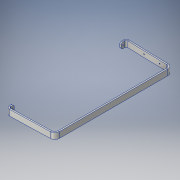
# Autodesk Inventor part: Panel_Strut
Saved by Autodesk Inventor 2016 (Build 200138000, 138)
## iProperties
Created: 2016-03-26
Part Number: Panel_Strut
Material: Aluminum 6061
Document SubType Name: Sheet Metal
Designer: agmle
Density: 2.7 g/cm^3
Sheet Metal Rule: Default
Appearance: Aluminum - Flat
Mass: 48.4378 g
Surface Area: 147.191 cm^2
Volume: 17.9399 cm^3
Flat Pattern Width: 1.27 cm
Flat Pattern Length: 46.2876 cm
Flat Pattern Area: 58.7853 cm^2
Sheet Metal Width: 0.500 in
Sheet Metal Length: 18.223 in
Sheet Metal Area: 9.112 in^2
Author: agmle
Autodesk Inventor part; units mm, degrees
ref_plane "YZ Plane" through (0, 0, 0) normal (1, 0, 0) x (0, 1, 0)
ref_plane "XZ Plane" through (0, 0, 0) normal (0, 1, 0) x (-1, 0, 0)
ref_plane "XY Plane" through (0, 0, 0) normal (0, 0, 1) x (1, 0, 0)
sketch "Sketch1" plane through (0, 0, 0) normal (0, 1, 0) x (-1, 0, 0)
  line L0 (110.8964, 130.0226) -> (9.5972, 127.37)
  line L1 (0, 117.5182) -> (0, -117.5182)
  line L2 (9.5972, -127.37) -> (110.8964, -130.0226)
  arc A0 (9.5972, 127.37) -> (0, 117.5182) centre (9.8552, 117.5182) ccw
  arc A1 (0, -117.5182) -> (9.5972, -127.37) centre (9.8552, -117.5182) ccw
  line L3 (110.8964, 130.0226) -> (0, 130.0226) construction
  line L4 (0, 130.0226) -> (0, -130.0226) construction
  line L5 (0, -130.0226) -> (110.8964, -130.0226) construction
  line L6 (110.8964, -130.0226) -> (110.8964, 130.0226) construction
  line L7 (102.7684, 130.0226) -> (102.7684, -130.0226) construction
  point P0 (0, 0)
  point P1 (0, 127.1187)
  point P2 (0, 0)
  dimension "d1" = 91.5
  dimension "d2" = 91.5
  dimension "d4" = 9.8552
  dimension "d15" = 260.0452
  dimension "d16" = 110.8964
  dimension "d17" = 8.128
  measures "d1" angle of L1 L0
  measures "d2" angle of L1 L2
  measures "d4" radius of A0
  measures "d15" distance of L5.end L3.start
  measures "d16" distance of L3.start L3.end
  measures "d17" distance between parallel lines of L6 L7
contour flange "Contour Flange1" sketch "Sketch1" thickness 3.048 bend radius 3.048 width 12.7 along (0, 1, 0) mid plane no both sides no wall seen from (-60.2468, 0, 128.6963) lies toward (-0.0261769, 0, -0.9996573) curves L0 A0 L1 A1 L2
bend "Bend1"
corner "Corner1"
sketch "Sketch2" plane through (-9.677, 0, 124.323) normal (-0.0261769, 0, -0.9996573) x (-0.9996573, 0, 0.0261769)
  line L0 (0, 0) -> (0, 12.7) construction
  line L1 (101.3339, 0) -> (0, 0) construction
  line L2 (101.3339, 12.7) -> (101.3339, 0) construction
  line L3 (0, 12.7) -> (101.3339, 12.7) construction
  line L4 (101.3339, 12.7) -> (0, 12.7) projected
  line L5 (90.1579, 12.7) -> (90.1579, 0)
  line L6 (101.3339, 0) -> (0, 0) projected
  point P0 (-12.9281, 0)
  dimension "d18" = 11.176
  constraints: 2 end point, 2 point on line, 1 perpendicular
  measures "d18" distance between parallel lines of L5 L2
sketch "Sketch3" plane through (-9.677, 0, -124.323) normal (-0.0261769, 0, 0.9996573) x (0.9996573, 0, 0.0261769)
  line L0 (0, 0) -> (0, 12.7) construction
  line L1 (-101.3339, 12.7) -> (0, 12.7) construction
  line L2 (-101.3339, 0) -> (-101.3339, 12.7) construction
  line L3 (0, 0) -> (-101.3339, 0) construction
  line L4 (-90.1579, 0) -> (-90.1579, 12.7)
  point P0 (12.9281, 0)
  dimension "d19" = 11.176
  constraints: 2 end point, 2 point on line, 1 perpendicular
  measures "d19" distance between parallel lines of L2 L4
fold "Fold1" angle 91.5 bend radius 3.048 thickness 3.048 k factor 0.44 line from (-99.804, 0, -126.6831) to (-99.804, 12.7, -126.6831) line at bend centre moving side (-0.9996573, 0, -0.0261769) folds toward (-0.0261769, 0, 0.9996573)
fold "Fold2" angle 91.5 bend radius 3.048 thickness 3.048 k factor 0.44 line from (-99.804, 12.7, 126.6831) to (-99.804, 0, 126.6831) line at bend centre moving side (-0.9996573, 0, 0.0261769) folds toward (-0.0261769, 0, -0.9996573)
sketch "Sketch4" plane through (-102.4763, 0, 123.5444) normal (-1, 0, 0) x (0, 0, 1)
  line L0 (0, 12.7) -> (0, 0) construction
  line L1 (0, 0) -> (-7.6713, 12.7) construction
  line L2 (-239.4174, 0) -> (-239.4174, 12.7) construction
  line L3 (-253.1848, 12.7) -> (-247.0888, 12.7) construction
  line L4 (-239.4174, 0) -> (-247.0888, 12.7) construction
  point P0 (-123.5444, 0)
  point P1 (-3.8357, 6.35)
  point P2 (-253.1827, 12.7)
  point P3 (-243.2531, 6.35)
  constraints: 4 end point, 2 midpoint
hole "Hole1" at (-102.4763, 6.35, 119.7087) at (-102.4763, 6.35, -119.7087) direction (1, 0, 0) diameter 2.159 depth 3.048
fillet "Corner Round1" radius 3.175 4 edges at (-100.9523, 12.7, -115.8731) (-100.9523, 0, -115.8731) (-100.9523, 12.7, 115.8731) (-100.9523, 0, 115.8731)
sketch "Sketch5" plane through (-9.5972, 0, -127.37) normal (0.0261769, 0, -0.9996573) x (-0.9996573, 0, -0.0261769)
  line L0 (0, 12.7) -> (86.6532, 12.7) projected
  line L1 (-9.8518, 12.7) -> (-9.8518, 0) projected
  point P0 (-12.9281, 0)
  point P1 (50.0922, 6.35)
  point P2 (15.5482, 6.35)
  dimension "d40" = 6.35
  dimension "d41" = 6.35
  dimension "d42" = 34.544
  dimension "d44" = 25.4
  measures "d40" distance from line of L0 point (50.092, 6.35)
  measures "d41" distance from line of L0 point (15.548, 6.35)
  measures "d42" distance of point (50.092, 6.35) point (15.548, 6.35)
  measures "d44" distance from line of L1 point (15.548, 6.35)
hole "Hole2" at (-59.6722, 6.35, -128.6812) at (-25.1401, 6.35, -127.777) direction (-0.0261769, 0, 0.9996573) diameter 2.159 end up to surface
equation "\"d2\" = d1"
equation "\"d4\" = Horizontal_Inside_Radius"
equation "\"d15\" = Inside_Height"
equation "\"d16\" = Inside_Depth"
equation "\"d17\" = Boss_Draft_Z"
equation "\"d18\" = Boss_Draft_Z + BendRadius"
equation "\"d19\" = Boss_Draft_Z + BendRadius"
equation "\"d20\" = BendReliefWidth"
equation "\"d21\" = BendReliefDepth"
equation "\"d22\" = MinimumRemnant"
equation "\"d23\" = BendRadius"
equation "\"d25\" = BendRadius"
equation "\"d26\" = BendReliefWidth"
equation "\"d27\" = BendReliefDepth"
equation "\"d28\" = MinimumRemnant"
equation "\"d29\" = BendRadius"
equation "\"d31\" = BendRadius"
equation "\"d37\" = Thickness"
equation "\"d5\" = BendReliefWidth"
equation "\"d6\" = BendReliefDepth"
equation "\"d7\" = MinimumRemnant"
equation "\"d8\" = BendRadius"
equation "\"d10\" = BendRadius"
equation "\"d12\" = CornerReliefSize"
equation "\"d13\" = GapSize"
equation "\"d14\" = JacobiRadiusSize"
equation "\"BendRadius\" = Thickness"
equation "\"BendReliefWidth\" = Thickness"
equation "\"BendReliefDepth\" = 0.5 * Thickness"
equation "\"CornerReliefSize\" = 4 * Thickness"
equation "\"MinimumRemnant\" = 2 * Thickness"
equation "\"TransitionRadius\" = BendRadius"
equation "\"JacobiRadiusSize\" = BendRadius"
equation "\"GapSize\" = Thickness"
equation "\"Horizontal_Inside_Radius\" = 9.8552"
equation "\"Inside_Height\" = 260.0452"
equation "\"Inside_Depth\" = 110.8964"
equation "\"Boss_Draft_Z\" = 8.128"
equation "\"Thickness\" = 3.048"
body "Solid1"
